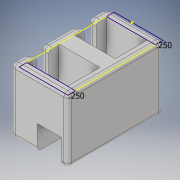
# Autodesk Inventor part: toggle_box
Saved by Autodesk Inventor 2018.1 (Build 221171000, 171)
## iProperties
Created: 2017-11-27
Part Number: toggle_box
Material: Generic
Document SubType Name: Modeling
Designer: bramd
Density: 1 g/cm^3
Appearance: Default
Author: bramd
Autodesk Inventor part; units mm, degrees
ref_plane "YZ Plane" through (0, 0, 0) normal (1, 0, 0) x (0, 1, 0)
ref_plane "XZ Plane" through (0, 0, 0) normal (0, 1, 0) x (-1, 0, 0)
ref_plane "XY Plane" through (0, 0, 0) normal (0, 0, 1) x (1, 0, 0)
sketch "Sketch1" plane through (0, 0, 0) normal (0, 0, 1) x (1, 0, 0)
  line L0 (0, 0) -> (20.066, 0)
  line L1 (20.066, 0) -> (20.066, 20.066)
  line L2 (20.066, 20.066) -> (0, 20.066)
  line L3 (0, 20.066) -> (0, 0)
  dimension "d0" = 20.066
  dimension "d1" = 20.066
  constraints: 8 end point, 2 parallel, 1 horizontal, 1 perpendicular
  measures "d0" distance of L2.end L1.end
  measures "d1" distance of L1.end L0.end
sketch "Sketch2" plane through (0, 0, 0) normal (0, 0, 1) x (1, 0, 0)
  line L0 (-5.08, 0) -> (25.146, 0)
  line L1 (25.146, 0) -> (25.146, 50.546)
  line L2 (25.146, 50.546) -> (-5.08, 50.546)
  line L3 (-5.08, 50.546) -> (-5.08, 0)
  point P0 (0, 0)
  dimension "d2" = 30.226
  dimension "d3" = 50.546
  constraints: 8 end point, 2 parallel, 1 horizontal, 1 perpendicular
  measures "d2" distance of L2.end L1.end
  measures "d3" distance of L1.end L0.end
extrude "Extrusion1" add sketch "Sketch2" along normal blind 78.74
extrude "Extrusion2" cut sketch "Sketch1" along normal blind 78.74
sketch "Sketch3" plane through (-5.08, 50.546, 0) normal (0, 1, 0) x (1, 0, 0)
  point P0 (5.08, 0)
sketch "Sketch4" plane through (-5.08, 50.546, 0) normal (0, 1, 0) x (1, 0, 0)
  point P0 (5.08, 0)
sketch "Sketch5" plane through (-5.08, 0, 0) normal (-1, 0, 0) x (0, 0, 1)
  line L0 (0, 0) -> (78.74, 0) projected
  line L1 (0, 50.546) -> (78.74, 50.546) projected
  line L2 (0, 0) -> (78.74, 0)
  line L3 (78.74, 0) -> (78.74, 50.546)
  line L4 (78.74, 50.546) -> (0, 50.546)
  line L5 (0, 50.546) -> (0, 0)
  constraints: 8 end point, 2 parallel, 1 horizontal, 1 perpendicular
extrude "Extrusion3" add sketch "Sketch5" along normal blind 10.16
sketch "Sketch6" plane through (25.146, 50.546, 78.74) normal (0, 1, 0) x (1, 0, 0)
  line L0 (-40.386, 78.74) -> (-40.386, 0) projected
  line L1 (0, 78.74) -> (0, 0) projected
  line L2 (-40.386, 78.74) -> (0, 78.74)
  line L3 (0, 78.74) -> (0, 72.39)
  line L4 (0, 72.39) -> (-40.386, 72.39)
  line L5 (-40.386, 72.39) -> (-40.386, 78.74)
  line L6 (-40.386, 0) -> (0, 0)
  line L7 (0, 0) -> (0, 6.35)
  line L8 (0, 6.35) -> (-40.386, 6.35)
  line L9 (-40.386, 6.35) -> (-40.386, 0)
  point P0 (-25.146, 78.74)
  dimension "d10" = 6.35
  dimension "d11" = 6.35
  constraints: 16 end point, 4 parallel, 2 horizontal, 2 perpendicular, 2 point on line
  measures "d10" distance of L2.end L3.end
  measures "d11" distance of L7.end L6.end
sketch "Sketch7" plane through (-15.24, 0, 0) normal (-1, 0, 0) x (0, 0, 1)
  line L0 (0, 0) -> (0, 50.546) projected
  line L1 (78.74, 20.066) -> (78.74, 0) projected
  line L2 (0, 50.546) -> (78.74, 50.546)
  line L3 (78.74, 50.546) -> (78.74, 0)
  line L4 (78.74, 0) -> (0, 0)
  line L5 (0, 0) -> (0, 50.546)
  constraints: 8 end point, 2 parallel, 1 horizontal, 1 perpendicular
extrude "Extrusion4" add sketch "Sketch7" along normal blind 6.35
sketch "Sketch8" plane through (25.146, 50.546, 78.74) normal (0, 1, 0) x (1, 0, 0)
  line L0 (-40.386, 6.35) -> (-6.35, 6.35)
  line L1 (-6.35, 6.35) -> (-6.35, 33.02)
  line L2 (-6.35, 33.02) -> (-40.386, 33.02)
  line L3 (-40.386, 33.02) -> (-40.386, 6.35)
  line L4 (-40.386, 45.7084) -> (-6.35, 45.7084)
  line L5 (-6.35, 45.7084) -> (-6.35, 72.3784)
  line L6 (-6.35, 72.3784) -> (-40.386, 72.3784)
  line L7 (-40.386, 72.3784) -> (-40.386, 45.7084)
  point P0 (-25.146, 78.74)
  dimension "d14" = 34.036
  dimension "d15" = 26.67
  dimension "d16" = 34.036
  dimension "d17" = 26.67
  constraints: 16 end point, 4 parallel, 2 horizontal, 2 perpendicular
  measures "d14" distance of L2.end L1.end
  measures "d15" distance of L1.end L0.end
  measures "d16" distance of L6.end L5.end
  measures "d17" distance of L5.end L5.start
sketch "Sketch9" plane through (0, 0, 0) normal (0, -1, 0) x (1, 0, 0)
  line L0 (-21.59, 0) -> (0, 0) projected
  line L1 (-21.59, 78.74) -> (-21.59, 0) projected
  line L2 (0, 0) -> (-21.59, 0)
  line L3 (-21.59, 0) -> (-21.59, 78.74)
  line L4 (-21.59, 78.74) -> (0, 78.74)
  line L5 (0, 78.74) -> (0, 0)
  line L6 (25.146, 0) -> (25.146, 78.74) projected
  line L7 (20.066, 78.74) -> (20.066, 0) projected
  line L8 (25.146, 78.74) -> (20.066, 78.74)
  line L9 (20.066, 78.74) -> (20.066, 0)
  line L10 (20.066, 0) -> (25.146, 0)
  line L11 (25.146, 0) -> (25.146, 78.74)
  constraints: 16 end point, 4 parallel, 2 horizontal, 2 perpendicular
extrude "Extrusion5" add sketch "Sketch9" along normal blind 2.54
sketch "Sketch10" plane through (0, 20.066, 0) normal (0, -1, 0) x (1, 0, 0)
  line L0 (20.066, 78.74) -> (0, 78.74)
  line L1 (0, 78.74) -> (0, 0)
  line L2 (0, 0) -> (20.066, 0)
  line L3 (20.066, 0) -> (20.066, 78.74)
  constraints: 8 end point, 2 parallel, 1 horizontal, 1 perpendicular
extrude "Extrusion6" add sketch "Sketch10" along normal blind 2.54
extrude "Extrusion7" cut sketch "Sketch8" against normal blind 31.75
sketch "Sketch11" plane through (25.146, 50.546, 78.74) normal (0, 1, 0) x (1, 0, 0)
  line L0 (-40.386, 6.35) -> (-40.386, 33.02) projected
  line L1 (-46.736, 0) -> (-46.736, 78.74) projected
  line L2 (-40.386, 14.605) -> (-46.736, 14.605)
  line L3 (-46.736, 14.605) -> (-46.736, 24.765)
  line L4 (-46.736, 24.765) -> (-40.386, 24.765)
  line L5 (-40.386, 24.765) -> (-40.386, 14.605)
  point P0 (-25.146, 78.74)
  dimension "d24" = 10.16
  constraints: 8 end point, 2 parallel, 2 point on line, 1 horizontal, 1 perpendicular
  measures "d24" distance of L2.end L3.end
sketch "Sketch12" plane through (25.146, 50.546, 78.74) normal (0, 1, 0) x (1, 0, 0)
  line L0 (-40.386, 45.7084) -> (-40.386, 72.3784) projected
  line L1 (-46.736, 0) -> (-46.736, 78.74) projected
  line L2 (-40.386, 64.1096) -> (-46.736, 64.1096)
  line L3 (-46.736, 64.1096) -> (-46.736, 53.9496)
  line L4 (-46.736, 53.9496) -> (-40.386, 53.9496)
  line L5 (-40.386, 53.9496) -> (-40.386, 64.1096)
  point P0 (-25.146, 78.74)
  dimension "d25" = 10.16
  constraints: 8 end point, 2 parallel, 2 point on line, 1 horizontal, 1 perpendicular
  measures "d25" distance of L3.end L2.end
extrude "Extrusion8" cut sketch "Sketch12" against normal blind 31.75
extrude "Extrusion9" cut sketch "Sketch11" against normal blind 31.75
fillet "Fillet1" radius 3.175 25 edges at (-21.59, 50.546, 71.4375) (-21.59, 50.546, 39.3827) (-21.59, 50.546, 7.3152) (-18.415, 50.546, 64.135) (-21.59, 34.671, 64.135) (-21.59, 34.671, 53.975) (-21.59, 34.671, 24.7904) (-21.59, 18.796, 19.7104) (-18.415, 50.546, 24.7904) (-18.415, 50.546, 53.975) (-18.415, 50.546, 14.6304) (-21.59, 34.671, 14.6304) (-21.59, 24.003, 0) (1.778, 50.546, 0) (-21.59, -2.54, 39.37) (-21.59, 24.003, 78.74) (1.778, 50.546, 78.74) (25.146, 24.003, 78.74) (22.606, -2.54, 78.74) (-10.795, -2.54, 78.74) (25.146, 50.546, 39.37) (25.146, 24.003, 0) (25.146, -2.54, 39.37) (-10.795, -2.54, 0) (22.606, -2.54, 0)
fillet "Fillet2" radius 3.175 2 edges at (-21.59, 18.796, 65.7225) (-21.59, 18.796, 52.3875)
body "Solid1"
